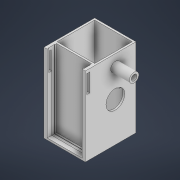
# Autodesk Inventor part: Measurement
Saved by Autodesk Inventor 2022 (Build 260153070, 153G)
## iProperties
Created: 2021-07-22
Part Number: Measurement
Material: Generic
Document SubType Name: Modeling
Designer: Eakawit_kor
Density: 1 g/cm^3
Appearance: Default
Author: Eakawit_kor
Autodesk Inventor part; units mm, degrees
ref_plane "YZ Plane" through (0, 0, 0) normal (1, 0, 0) x (0, 1, 0)
ref_plane "XZ Plane" through (0, 0, 0) normal (0, 1, 0) x (-1, 0, 0)
ref_plane "XY Plane" through (0, 0, 0) normal (0, 0, 1) x (1, 0, 0)
sketch "Sketch1" plane through (0, 0, 0) normal (0, 0, 1) x (1, 0, 0)
  line L0 (0, 0) -> (22, 0)
  line L1 (22, 0) -> (22, 42)
  line L2 (22, 42) -> (0, 42)
  line L3 (0, 42) -> (0, 0)
  dimension "d0" = 42
  dimension "d1" = 22
  constraints: 8 end point, 2 parallel, 1 horizontal, 1 perpendicular
  measures "d0" distance of L2.end L0.start
  measures "d1" distance of L1.end L2.end
extrude "Extrusion1" add sketch "Sketch1" along normal blind 22
sketch "Sketch2" plane through (0, 0, 0) normal (-1, 0, 0) x (0, 0, 1)
  circle A0 centre (11, 5) radius 2.5
  line L0 (0, 42) -> (0, 0) projected
  line L1 (0, 0) -> (22, 0) projected
  dimension "d4" = 11
  dimension "d5" = 5
  dimension "d6" = 5
  constraints: 1 centre point
  measures "d4" distance from line of L0 A0.centre
  measures "d5" diameter of A0
  measures "d6" distance from line of L1 A0.centre
extrude "Extrusion2" add sketch "Sketch2" along normal blind 10
sketch "Sketch3" plane through (22, 0, 0) normal (1, 0, 0) x (0, 0, -1)
  circle A0 centre (-11, 36) radius 2.5
  line L0 (0, 42) -> (-22, 42) projected
  line L1 (0, 0) -> (0, 42) projected
  dimension "d9" = 5
  dimension "d10" = 6
  dimension "d11" = 11
  constraints: 1 centre point
  measures "d9" diameter of A0
  measures "d10" distance from line of L0 A0.centre
  measures "d11" distance from line of L1 A0.centre
extrude "Extrusion3" add sketch "Sketch3" along normal blind 10
sketch "Sketch4" plane through (0, 42, 0) normal (0, 1, 0) x (1, 0, 0)
  line L0 (1, -1) -> (21, -1)
  line L1 (21, -1) -> (21, -21)
  line L2 (21, -21) -> (1, -21)
  line L3 (1, -21) -> (1, -1)
  line L4 (0, 0) -> (0, -22) projected
  line L5 (22, 0) -> (0, 0) projected
  line L6 (22, 0) -> (22, -22) projected
  line L7 (22, -22) -> (0, -22) projected
  dimension "d14" = 1
  dimension "d15" = 1
  dimension "d16" = 1
  dimension "d17" = 1
  constraints: 8 end point, 2 parallel, 1 horizontal, 1 perpendicular
  measures "d14" distance between parallel lines of L4 L3
  measures "d15" distance between parallel lines of L5 L0
  measures "d16" distance between parallel lines of L6 L1
  measures "d17" distance between parallel lines of L7 L2
extrude "Extrusion4" cut sketch "Sketch4" against normal blind 41 contours L0 L1 L2 L3
sketch "Sketch5" plane through (0, 0, 0) normal (-1, 0, 0) x (0, 0, 1)
  circle A0 centre (11, 21) radius 5
  line L0 (0, 42) -> (0, 0) projected
  line L1 (0, 0) -> (22, 0) projected
  dimension "d20" = 11
  dimension "d21" = 10
  dimension "d22" = 21
  constraints: 1 centre point
  measures "d20" distance from line of L0 A0.centre
  measures "d21" diameter of A0
  measures "d22" distance from line of L1 A0.centre
extrude "Extrusion5" cut sketch "Sketch5" against normal through all
sketch "Sketch6" plane through (0, 0, 0) normal (0, 0, -1) x (-1, 0, 0)
  circle A0 centre (-11, 21) radius 5
  line L0 (0, 0) -> (-22, 0) projected
  line L1 (0, 42) -> (0, 0) projected
  dimension "d25" = 21
  dimension "d26" = 11
  dimension "d27" = 10
  constraints: 1 centre point
  measures "d25" distance from line of L0 A0.centre
  measures "d26" distance from line of L1 A0.centre
  measures "d27" diameter of A0
extrude "Extrusion6" cut sketch "Sketch6" against normal up to surface (1 mm away)
sketch "Sketch7" plane through (-10, 5, 11) normal (-1, 0, 0) x (0, 0, 1)
  circle A0 centre (0, 0) radius 1.5
  circle A1 centre (0, 0) radius 2.5 projected
  point P0 (-11, -5)
  dimension "d30" = 1
  constraints: 1 centre point, 1 concentric
  measures "d30" radial gap between concentric circles of A1 A0
extrude "Extrusion7" cut sketch "Sketch7" against normal up to surface (11 mm away) contours A0
sketch "Sketch8" plane through (32, 36, 11) normal (1, 0, 0) x (0, 0, -1)
  circle A0 centre (0, 0) radius 1.5
  circle A1 centre (0, 0) radius 2.5 projected
  point P0 (11, -36)
  dimension "d33" = 1
  constraints: 1 centre point, 1 concentric
  measures "d33" radial gap between concentric circles of A1 A0
extrude "Extrusion8" cut sketch "Sketch8" against normal up to surface (11 mm away) contours A0
sketch "Sketch9" plane through (0, 0, 22) normal (0, 0, 1) x (1, 0, 0)
  line L0 (20.3, 42) -> (20.3, 1)
  line L1 (20.3, 1) -> (1.7, 1)
  line L2 (1.7, 1) -> (1.7, 42)
  line L3 (0, 42) -> (0, 0) projected
  line L4 (0, 0) -> (22, 0) projected
  line L5 (22, 42) -> (0, 42) projected
  line L6 (22, 42) -> (0, 42) projected
  line L7 (1.7, 42) -> (0, 42)
  line L8 (0, 42) -> (0, 0) projected
  line L9 (0, 42) -> (0, 0)
  line L10 (0, 0) -> (22, 0)
  line L11 (22, 0) -> (22, 42) projected
  line L12 (22, 0) -> (22, 42)
  line L13 (22, 0) -> (22, 42) projected
  line L14 (20.3, 42) -> (22, 42)
  point P0 (1.7, 42)
  dimension "d37" = 1.7
  dimension "d38" = 1
  constraints: 16 end point, 3 perpendicular, 2 collinear, 1 parallel, 1 vertical
  measures "d37" distance between parallel lines of L3 L2
  measures "d38" distance between parallel lines of L4 L1
extrude "Extrusion9" add sketch "Sketch9" along normal blind 5 contours L5 L11 L4 L3 L2 L1 L0
sketch "Sketch10" plane through (0, 42, 0) normal (0, 1, 0) x (1, 0, 0)
  line L0 (20.5, -24.6) -> (1.5, -24.6)
  line L1 (1.5, -24.6) -> (1.5, -23)
  line L2 (1.5, -23) -> (20.5, -23)
  line L3 (20.5, -23) -> (20.5, -24.6)
  line L4 (0, 0) -> (0, -27) projected
  line L5 (20.3, -22) -> (1.7, -22) projected
  dimension "d41" = 19
  dimension "d42" = 1.6
  dimension "d43" = 1.5
  dimension "d44" = 1
  constraints: 8 end point, 2 parallel, 1 horizontal, 1 perpendicular
  measures "d41" distance of L0.start L0.end
  measures "d42" distance of L2.end L0.start
  measures "d43" distance between parallel lines of L4 L1
  measures "d44" distance between parallel lines of L5 L2
extrude "Extrusion10" cut sketch "Sketch10" against normal blind 41.2
sketch "Sketch12" plane through (1.7, 1, 27) normal (1, 0, 0) x (0, 0, -1)
  line L0 (2.4, 41) -> (2.4, -0.2) projected
  line L1 (2.4, 39.39) -> (0.9, 39.39)
  line L2 (0.9, 39.39) -> (0.9, 29.74)
  line L3 (0.9, 29.74) -> (2.4, 29.74)
  line L4 (2.4, 29.74) -> (2.4, 39.39)
  line L5 (2.4, -0.2) -> (4, -0.2) projected
  point P0 (27, -1)
  point P1 (2.4, 29.74)
  dimension "d48" = 1.5
  dimension "d49" = 9.65
  dimension "d50" = 29.94
  constraints: 8 end point, 2 parallel, 1 horizontal, 1 perpendicular, 1 point on line
  measures "d48" distance of L1.start L1.end
  measures "d49" distance of L1.end L2.end
  measures "d50" distance between parallel lines of L5 L3
extrude "Extrusion11" cut sketch "Sketch12" along normal through all both and the other way through all
sketch "Sketch13" plane through (20.3, 1, 27) normal (-1, 0, 0) x (0, 0, 1)
  line L0 (-2.4, 39.39) -> (-2.4, 29.74) projected
  line L1 (-2.4, 39.39) -> (-0.9, 39.39)
  line L2 (-0.9, 39.39) -> (-0.9, 41)
  line L3 (-0.9, 41) -> (-2.4, 41)
  line L4 (-2.4, 41) -> (-2.4, 39.39)
  line L5 (-0.9, 39.39) -> (-0.9, 29.74) projected
  line L6 (-2.4, 41) -> (0, 41) projected
  point P0 (-27, -1)
  constraints: 8 end point, 2 collinear, 2 parallel, 1 horizontal, 1 perpendicular
extrude "Extrusion12" cut sketch "Sketch13" against normal up to surface (0.2 mm away)
sketch "Sketch14" plane through (1.7, 1, 27) normal (1, 0, 0) x (0, 0, -1)
  line L0 (2.4, 39.39) -> (2.4, 41) projected
  line L1 (2.4, 39.39) -> (0.9, 39.39)
  line L2 (0.9, 39.39) -> (0.9, 41)
  line L3 (0.9, 41) -> (2.4, 41)
  line L4 (2.4, 41) -> (2.4, 39.39)
  line L5 (0.9, 29.74) -> (0.9, 39.39) projected
  line L6 (2.4, 41) -> (0, 41) projected
  point P0 (27, -1)
  constraints: 8 end point, 2 collinear, 2 parallel, 1 horizontal, 1 perpendicular
extrude "Extrusion13" cut sketch "Sketch14" against normal up to surface (0.2 mm away)
body "Solid1"
